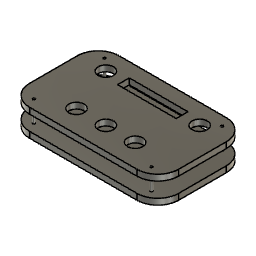
HyperShades Console mk.1 (Autodesk Fusion 360 design; units mm, degrees)
Autodesk Fusion 360 part; units mm, degrees
sketch "TopSketch" plane through (0, 0, 0) normal (0, 0, 1) x (1, 0, 0)
  line L0 (45.72, 38.1) -> (-45.72, 38.1)
  line L1 (-63.5, 20.32) -> (-63.5, -20.32)
  line L2 (-45.72, -38.1) -> (45.72, -38.1)
  line L3 (63.5, -20.32) -> (63.5, 20.32)
  line L4 (63.5, 38.1) -> (-63.5, -38.1) construction
  line L5 (-63.5, 38.1) -> (63.5, -38.1) construction
  arc A0 (-45.72, 38.1) -> (-63.5, 20.32) centre (-45.72, 20.32) ccw
  arc A1 (-63.5, -20.32) -> (-45.72, -38.1) centre (-45.72, -20.32) ccw
  arc A2 (45.72, -38.1) -> (63.5, -20.32) centre (45.72, -20.32) ccw
  arc A3 (63.5, 20.32) -> (45.72, 38.1) centre (45.72, 20.32) ccw
  line L6 (-25, 26.1) -> (25, 26.1)
  line L7 (25, 26.1) -> (25, 16.1)
  line L8 (25, 16.1) -> (-25, 16.1)
  line L9 (-25, 16.1) -> (-25, 26.1)
  circle A4 centre (40, 21.1) radius 6.5
  circle A5 centre (25, -18.9) radius 6.5
  circle A6 centre (0, -18.9) radius 6.5
  line L10 (0, 38.1) -> (0, -38.1) construction
  circle A7 centre (-40, 21.1) radius 6.5
  circle A8 centre (-25, -18.9) radius 6.5
  line L11 (61.2418, 9.5468) -> (17.2418, 9.5468)
  line L12 (17.2418, 9.5468) -> (17.2418, -9.4532)
  line L13 (17.2418, -9.4532) -> (61.2418, -9.4532)
  line L14 (61.2418, -9.4532) -> (61.2418, 9.5468)
  line L15 (61.2418, 9.5468) -> (17.2418, -9.4532) construction
  line L16 (17.2418, 9.5468) -> (61.2418, -9.4532) construction
  point P0 (0, 26.1)
  point P1 (-25, 21.1)
  point P2 (25, 21.1)
  point P3 (39.2418, 0.0468)
  dimension "d1" = 127
  dimension "d2" = 76.2
  dimension "d3" = 17.78
  dimension "d4" = 17.78
  dimension "d5" = 17.78
  dimension "d6" = 17.78
  dimension "d10" = 50
  dimension "d11" = 10
  dimension "d12" = 13
  dimension "d13" = 12
  dimension "d14" = 15
  dimension "d15" = 13
  dimension "d16" = 35
  dimension "d17" = 13
  dimension "d28" = 44
  dimension "d29" = 19
  constraint horizontal L0
  constraint perpendicular L0 L1
  constraint parallel L0 L2
  constraint parallel L1 L3
  constraint coincident L4 origin
  constraint coincident L5 origin
  constraint coincident L5.start L0
  constraint coincident L5.start L1
  constraint tangent L0 A0
  constraint tangent L1 A0
  constraint coincident L4.end L2
  constraint coincident L4.end L1
  constraint tangent L2 A1
  constraint tangent L1 A1
  constraint coincident L5.end L2
  constraint coincident L5.end L3
  constraint tangent L2 A2
  constraint tangent L3 A2
  constraint coincident L4.start L0
  constraint coincident L4.start L3
  constraint tangent L0 A3
  constraint tangent L3 A3
  constraint horizontal L6
  constraint vertical L7
  constraint horizontal L8
  constraint vertical L9
  constraint midpoint L6 P0
  constraint vertical origin P0
  constraint midpoint L9 P1
  constraint midpoint L7 P2
  constraint horizontal A4.centre P2
  constraint vertical L7.end A5.centre
  constraint horizontal A5.centre A6.centre
  constraint vertical origin A6.centre
  constraint perpendicular L2 L10
  constraint coincident L2 L10.end
  constraint coincident L0 L10.start
  constraint vertical origin L10.start
  constraint symmetric A4 L10 A7
  constraint symmetric A5 L10 A8
  constraint horizontal L11
  constraint perpendicular L11 L12
  constraint parallel L11 L13
  constraint parallel L12 L14
  constraint coincident L15 P3
  constraint coincident L16 P3
  measures "d1" distance of L4.end L5.end
  measures "d2" distance of L5.start L4.end
  measures "d3" radius of A0
  measures "d4" radius of A1
  measures "d5" radius of A2
  measures "d6" radius of A3
  measures "d10" distance of L6.start L6.end
  measures "d11" distance of L6.start L8.end
  measures "d12" diameter of A4
  measures "d13" distance of L0 P0
  measures "d14" distance of A4.centre P2
  measures "d15" diameter of A5
  measures "d16" distance of L7.end A5.centre
  measures "d17" diameter of A6
  measures "d28" distance of L12.end L13.end
  measures "d29" distance of L11.end L12.end
extrude "Extrude1" add sketch "TopSketch" along normal blind 5.08 contours L0 L1 L2 L3 A0 A1 A2 A3 | L11 L12 L13 L14 makes body 1
sketch "StandSketch" plane through (0, 0, 0) normal (0, 0, -1) x (1, 0, 0)
  circle A0 centre (-25, 18.9) radius 6.5
  circle A1 centre (25, 18.9) radius 6.5
  circle A2 centre (0, 18.9) radius 6.5
  circle A3 centre (-40, -21.1) radius 6.5
  circle A4 centre (40, -21.1) radius 6.5
  line L0 (-25, -16.1) -> (25, -16.1)
  line L1 (25, -16.1) -> (25, -26.1)
  line L2 (25, -26.1) -> (-25, -26.1)
  line L3 (-25, -26.1) -> (-25, -16.1)
  arc A5 (45.72, -38.1) -> (63.5, -20.32) centre (45.72, -20.32) ccw
  line L4 (63.5, -20.32) -> (63.5, 20.32)
  arc A6 (63.5, 20.32) -> (45.72, 38.1) centre (45.72, 20.32) ccw
  line L5 (45.72, 38.1) -> (-45.72, 38.1)
  arc A7 (-45.72, 38.1) -> (-63.5, 20.32) centre (-45.72, 20.32) ccw
  line L6 (-63.5, 20.32) -> (-63.5, -20.32)
  arc A8 (-63.5, -20.32) -> (-45.72, -38.1) centre (-45.72, -20.32) ccw
  line L7 (-45.72, -38.1) -> (45.72, -38.1)
  line L8 (63.5, 38.1) -> (-63.5, 38.1) construction
  line L9 (-63.5, 38.1) -> (-63.5, -38.1) construction
  line L10 (-63.5, -38.1) -> (63.5, -38.1) construction
  line L11 (63.5, -38.1) -> (63.5, 38.1) construction
  line L12 (63.5, 38.1) -> (-63.5, -38.1) construction
  line L13 (-63.5, 38.1) -> (63.5, -38.1) construction
  circle A9 centre (-50.1667, 30.1) radius 1.016
  line L14 (0, 38.1) -> (0, -38.1) construction
  line L15 (-63.5, 0) -> (63.5, 0) construction
  circle A10 centre (50.1667, 30.1) radius 1.016
  circle A11 centre (-50.1667, -30.1) radius 1.016
  circle A12 centre (50.1667, -30.1) radius 1.016
  dimension "d18" = 127
  dimension "d19" = 76.2
  dimension "d20" = 2.032
  dimension "d21" = 8
  constraint horizontal L8
  constraint perpendicular L8 L9
  constraint parallel L8 L10
  constraint parallel L9 L11
  constraint coincident L12 origin
  constraint coincident L13 origin
  constraint coincident L13 A9.centre
  constraint midpoint L8 L14.start
  constraint midpoint L10 L14.end
  constraint midpoint L9 L15.start
  constraint midpoint L11 L15.end
  constraint symmetric A9 L14 A10
  constraint symmetric A9 L15 A11
  constraint symmetric L15 A10 A12
  measures "d18" distance of L9.end L10.end
  measures "d19" distance of L8.end L9.end
  measures "d20" diameter of A9
  measures "d21" distance of L8 A9.centre
extrude "Extrude3" add sketch "StandSketch" along normal blind 12.7 separate body contours A9 | A10 | A11 | A12 makes body 2 at (50.1413, -31.1157, -8.4667) makes body 3 at (50.1413, 29.0843, -8.4667) makes body 4 at (-50.192, -31.1157, -8.4667) makes body 5 at (-50.192, 29.0843, -8.4667)
extrude "Extrude2" cut sketch "StandSketch" against normal up to surface (5.08 mm away) contours A9 | A10 | A11 | A12 bodies 1
sketch "BotSketch" plane through (0, 0, -12.7) normal (0, 0, -1) x (1, 0, 0)
  circle A0 centre (50.1667, 30.1) radius 1.016
  circle A1 centre (-50.1667, -30.1) radius 1.016
  circle A2 centre (50.1667, -30.1) radius 1.016
  circle A3 centre (-50.1667, 30.1) radius 1.016
  circle A4 centre (50.1667, 30.1) radius 1.016
  circle A5 centre (-25, 18.9) radius 6.5
  circle A6 centre (25, 18.9) radius 6.5
  circle A7 centre (0, 18.9) radius 6.5
  circle A8 centre (-40, -21.1) radius 6.5
  circle A9 centre (40, -21.1) radius 6.5
  line L0 (-25, -16.1) -> (25, -16.1)
  line L1 (25, -16.1) -> (25, -26.1)
  line L2 (25, -26.1) -> (-25, -26.1)
  line L3 (-25, -26.1) -> (-25, -16.1)
  arc A10 (45.72, -38.1) -> (63.5, -20.32) centre (45.72, -20.32) ccw
  line L4 (63.5, -20.32) -> (63.5, 20.32)
  arc A11 (63.5, 20.32) -> (45.72, 38.1) centre (45.72, 20.32) ccw
  line L5 (45.72, 38.1) -> (-45.72, 38.1)
  arc A12 (-45.72, 38.1) -> (-63.5, 20.32) centre (-45.72, 20.32) ccw
  line L6 (-63.5, 20.32) -> (-63.5, -20.32)
  arc A13 (-63.5, -20.32) -> (-45.72, -38.1) centre (-45.72, -20.32) ccw
  line L7 (-45.72, -38.1) -> (45.72, -38.1)
extrude "Extrude4" add sketch "BotSketch" along normal blind 5.08 separate body contours A5 | A6 | A7 | A8 | A9 | L0 L1 L2 L3 | A10 L4 A11 L5 A12 L6 A13 L7 makes body 6
sketch "Sketch4" plane through (0, 0, 5.08) normal (0, 0, 1) x (-1, 0, 0)
  circle A0 centre (50.1667, -30.1) radius 1.016
  circle A1 centre (-50.1667, -30.1) radius 1.016
  circle A2 centre (50.1667, 30.1) radius 1.016
  circle A3 centre (-50.1667, 30.1) radius 1.016
  circle A4 centre (25, 18.9) radius 6.5
  circle A5 centre (40, -21.1) radius 6.5
  circle A6 centre (0, 18.9) radius 6.5
  circle A7 centre (-25, 18.9) radius 6.5
  circle A8 centre (-40, -21.1) radius 6.5
  line L0 (-25, -16.1) -> (25, -16.1)
  line L1 (25, -16.1) -> (25, -26.1)
  line L2 (25, -26.1) -> (-25, -26.1)
  line L3 (-25, -26.1) -> (-25, -16.1)
  arc A9 (-63.5, -20.32) -> (-45.72, -38.1) centre (-45.72, -20.32) ccw
  line L4 (-45.72, -38.1) -> (45.72, -38.1)
  arc A10 (45.72, -38.1) -> (63.5, -20.32) centre (45.72, -20.32) ccw
  line L5 (63.5, -20.32) -> (63.5, 20.32)
  arc A11 (63.5, 20.32) -> (45.72, 38.1) centre (45.72, 20.32) ccw
  line L6 (45.72, 38.1) -> (-45.72, 38.1)
  arc A12 (-45.72, 38.1) -> (-63.5, 20.32) centre (-45.72, 20.32) ccw
  line L7 (-63.5, 20.32) -> (-63.5, -20.32)
sketch "Sketch5" plane through (0, 0, -17.78) normal (0, 0, -1) x (1, 0, 0)
  circle A0 centre (50.1667, -30.1) radius 1.016
  circle A1 centre (50.1667, 30.1) radius 1.016
  circle A2 centre (-50.1667, 30.1) radius 1.016
  circle A3 centre (-50.1667, -30.1) radius 1.016
  line L0 (-45.72, -38.1) -> (45.72, -38.1)
  arc A4 (45.72, -38.1) -> (63.5, -20.32) centre (45.72, -20.32) ccw
  line L1 (63.5, -20.32) -> (63.5, 20.32)
  arc A5 (63.5, 20.32) -> (45.72, 38.1) centre (45.72, 20.32) ccw
  line L2 (45.72, 38.1) -> (-45.72, 38.1)
  arc A6 (-45.72, 38.1) -> (-63.5, 20.32) centre (-45.72, 20.32) ccw
  line L3 (-63.5, 20.32) -> (-63.5, -20.32)
  arc A7 (-63.5, -20.32) -> (-45.72, -38.1) centre (-45.72, -20.32) ccw
equation "matThickness = 0.2 in"
equation "d8 = matThickness"
equation "d26 = matThickness"
named bodies: "Top", "Standoff(1)", "Standoff(2)", "Standoff(3)", "Standoff(4)", "Base"
